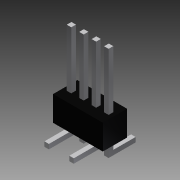
# Autodesk Inventor part: Header_127
Saved by Autodesk Inventor 2014 (Build 180170000, 170)
## iProperties
Created: 2015-11-05
Part Number: Header_127
Material: Generic
Document SubType Name: Modeling
Designer: Owner
Density: 1 g/cm^3
Appearance: Default
Author: Owner
Autodesk Inventor part; units mm, degrees
ref_plane "YZ Plane" through (0, 0, 0) normal (1, 0, 0) x (0, 1, 0)
sketch "Sketch1" plane through (0, 0, 0) normal (0, 1, 0) x (-1, 0, 0)
  line L0 (-2.7896, 0.599) -> (2.2904, 0.599)
  line L1 (2.2904, 0.599) -> (2.2904, -1.881)
  line L2 (2.2904, -1.881) -> (-2.7896, -1.881)
  line L3 (-2.7896, -1.881) -> (-2.7896, 0.599)
  point P0 (0, 0)
  dimension "d0" = 5.08
  dimension "d1" = 2.48
  constraints: 8 end point, 2 parallel, 1 horizontal, 1 perpendicular
  measures "d0" distance of L0.start L0.end
  measures "d1" distance of L0.end L1.end
extrude "Extrusion1" add sketch "Sketch1" along normal blind 2.54
ref_plane "Work Plane1" through (2.1546, 0, 0.599) normal (1, 0, 0) x (0, 0, -1)
sketch "Sketch2" plane through (2.1546, 0, 0.599) normal (1, 0, 0) x (0, 0, -1)
  line L0 (0.99, 8.38) -> (1.47, 8.38)
  line L1 (1.47, 8.38) -> (1.47, -0.79)
  line L2 (0.99, -0.142) -> (0.99, 8.38)
  line L3 (3.75, -0.79) -> (1.47, -0.79)
  line L4 (0.99, -0.142) -> (0.99, -1.27)
  line L5 (0.99, -1.27) -> (3.75, -1.27)
  line L6 (3.75, -1.27) -> (3.75, -0.79)
  line L7 (0, 2.54) -> (2.48, 2.54) projected
  line L8 (2.48, 0) -> (0, 0) projected
  line L9 (2.48, 0) -> (2.48, 2.54) projected
  point P0 (0.599, 0)
  dimension "d5" = 0.48
  dimension "d6" = 0.48
  dimension "d7" = 5.84
  dimension "d8" = 1.27
  dimension "d9" = 1.01
  dimension "d10" = 1.27
  constraints: 14 end point, 3 parallel, 2 horizontal, 2 perpendicular
  measures "d5" distance of L5.end L3.start
  measures "d6" distance of L0.start L0.end
  measures "d7" distance between parallel lines of L7 L0
  measures "d8" distance between parallel lines of L5 L8
  measures "d9" distance between parallel lines of L9 L1
  measures "d10" distance between parallel lines of L6 L9
extrude "Extrusion2" add sketch "Sketch2" along normal mid plane 0.46 contours L0 L1 L7 L2 | L7 L1 L8 L2 | L8 L1 L3 L6 L5 L4 L2
pattern_linear "Rectangular Pattern1" count 2 spacing 2.54 along (-1, 0, 0) of "Extrusion2"
ref_plane "Work Plane2" through (0.8846, 0, 0.599) normal (1, 0, 0) x (0, 0, -1)
sketch "Sketch3" plane through (0.8846, 0, 0.599) normal (1, 0, 0) x (0, 0, -1)
  line L0 (0.99, 8.38) -> (1.47, 8.38)
  line L1 (1.47, 8.38) -> (1.47, -0.79)
  line L2 (0.99, -0.142) -> (0.99, 8.38)
  line L3 (0.99, -0.142) -> (0.99, -0.79)
  line L4 (1.47, 8.38) -> (0.99, 8.38)
  line L5 (0.99, 8.38) -> (0.99, -0.79)
  line L6 (1.47, -0.142) -> (1.47, 8.38)
  line L7 (-1.29, -0.79) -> (0.99, -0.79)
  line L8 (1.47, -0.142) -> (1.47, -1.27)
  line L9 (1.47, -1.27) -> (-1.29, -1.27)
  line L10 (-1.29, -1.27) -> (-1.29, -0.79)
  point P0 (0.599, 0)
  dimension "d18" = 0.48
  constraints: 22 end point, 1 horizontal, 1 parallel, 1 perpendicular
  measures "d18" distance of L0.start L0.end
extrude "Extrusion3" add sketch "Sketch3" along normal mid plane 0.46
pattern_linear "Rectangular Pattern2" count 2 spacing 2.54 along (-1, 0, 0) of "Extrusion3"
body "Solid1"
